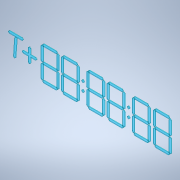
# Autodesk Inventor part: LED Clock Lights
Saved by Autodesk Inventor 2021 (Build 250183000, 183)
## iProperties
Created: 2020-06-27
Part Number: LED Clock Lights
Material: LED Bright
Document SubType Name: Modeling
Designer: dech3
Density: 1.188 g/cm^3
Appearance: Polycarbonate - Clear(2)
Author: dech3
Autodesk Inventor part; units mm, degrees
(part 1 of 2)
ref_plane "YZ Plane" through (0, 0, 0) normal (1, 0, 0) x (0, 1, 0)
ref_plane "XZ Plane" through (0, 0, 0) normal (0, 1, 0) x (-1, 0, 0)
ref_plane "XY Plane" through (0, 0, 0) normal (0, 0, 1) x (1, 0, 0)
sketch "Dot" plane through (0, 0, 0) normal (0, 0, 1) x (1, 0, 0)
  line L0 (-34.9663, 29.5091) -> (-32.9663, 29.5091)
  line L1 (-32.9663, 29.5091) -> (-29.7663, 26.3091)
  line L2 (-29.7663, 26.3091) -> (-29.7663, 24.3091)
  line L3 (-29.7663, 24.3091) -> (-32.9663, 21.1091)
  line L4 (-32.9663, 21.1091) -> (-34.9663, 21.1091)
  line L5 (-34.9663, 21.1091) -> (-38.1663, 24.3091)
  line L6 (-38.1663, 24.3091) -> (-38.1663, 26.3091)
  line L7 (-38.1663, 26.3091) -> (-34.9663, 29.5091)
  point P0 (-33.9663, 25.3091)
  dimension "d88" = 0
  dimension "d89" = 0
  dimension "d90" = 0
  dimension "d91" = 0
  dimension "d92" = 10
  dimension "d93" = 7.5
  dimension "d94" = 25
  dimension "d95" = 7.5
  dimension "d96" = 25
  dimension "d97" = 1.1
  dimension "d98" = 21
  dimension "d99" = 21
  dimension "d100" = 21
  dimension "d101" = 0
  dimension "d102" = 21
  dimension "d103" = 21
  dimension "d104" = 0
  dimension "d105" = 21
  dimension "d106" = 39
  dimension "d107" = 0
  dimension "d108" = 18
  dimension "d109" = 23
  dimension "d110" = 11.5
  dimension "d111" = 11.5
  dimension "d0" = 3.2
  dimension "d1" = 3.2
  dimension "d2" = 3.2
  dimension "d3" = 3.2
  dimension "d4" = 3.2
  dimension "d5" = 3.2
  dimension "d6" = 3.2
  dimension "d7" = 3.2
  dimension "d8" = 2
  dimension "d9" = 2
  dimension "d10" = 2
  dimension "d11" = 2
  measures "d0" horizontal distance of L1.end L0.end
  measures "d1" horizontal distance of L0.start L6.end
  measures "d2" horizontal distance of L0.start L6.end
  measures "d3" horizontal distance of L1.end L0.end
  measures "d4" horizontal distance of L4.end L5.end
  measures "d5" horizontal distance of L2.end L3.end
  measures "d6" horizontal distance of L2.end L3.end
  measures "d7" horizontal distance of L5.end L4.end
  measures "d8" distance of L1.end L2.end
  measures "d9" distance of L0.end L0.start
  measures "d10" distance of L3.end L4.end
  measures "d11" distance of L6.end L5.end
sketch "Slanted Segment Large" plane through (0, 0, 0) normal (0, 0, 1) x (1, 0, 0)
  line L0 (-252.8296, -124.6537) -> (-254.4296, -124.6537)
  line L1 (-254.4296, -124.6537) -> (-257.6296, -127.8537)
  line L2 (-257.6296, -127.8537) -> (-261.6917, -184.8537)
  line L3 (-253.6917, -184.8537) -> (-249.6296, -127.8537)
  line L4 (-249.6296, -127.8537) -> (-252.8296, -124.6537)
  line L5 (-261.6917, -184.8537) -> (-258.4917, -188.0537)
  line L6 (-258.4917, -188.0537) -> (-256.8917, -188.0537)
  line L7 (-256.8917, -188.0537) -> (-253.6917, -184.8537)
  point P0 (-253.3255, -154.094)
  point P1 (-253.6296, -124.6537)
  dimension "d88" = 0
  dimension "d89" = 0
  dimension "d90" = 0
  dimension "d91" = 0
  dimension "d92" = 10
  dimension "d93" = 7.5
  dimension "d94" = 25
  dimension "d95" = 7.5
  dimension "d96" = 25
  dimension "d97" = 1.1
  dimension "d98" = 21
  dimension "d99" = 21
  dimension "d100" = 21
  dimension "d101" = 0
  dimension "d102" = 21
  dimension "d103" = 21
  dimension "d104" = 0
  dimension "d105" = 21
  dimension "d106" = 39
  dimension "d107" = 0
  dimension "d108" = 18
  dimension "d109" = 23
  dimension "d110" = 11.5
  dimension "d111" = 11.5
  dimension "d12" = 3.2
  dimension "d13" = 3.2
  dimension "d14" = 8
  dimension "d15" = 3.2
  dimension "d16" = 3.2
  dimension "d17" = 57
  dimension "d18" = 3.2
  dimension "d19" = 3.2
  dimension "d20" = 3.2
  dimension "d21" = 3.2
  measures "d12" horizontal distance of L0.end L1.end
  measures "d13" horizontal distance of L3.end L0.start
  measures "d14" distance of L3.end L1.end
  measures "d15" horizontal distance of L3.end L0.start
  measures "d16" horizontal distance of L0.end L1.end
  measures "d17" vertical distance of L3.end L3.start
  measures "d18" horizontal distance of L5.end L2.end
  measures "d19" horizontal distance of L3.start L6.end
  measures "d20" horizontal distance of L2.end L5.end
  measures "d21" horizontal distance of L3.start L6.end
sketch "Single Segment" plane through (0, 0, 0) normal (0, 0, 1) x (1, 0, 0)
  arc A0 (130.9839, -3.9071) -> (131.691, -4.2) centre (131.691, -3.2) ccw
  arc A1 (131.691, 3.8) -> (130.9839, 3.5071) centre (131.691, 2.8) ccw
  line L0 (130.9839, -3.9071) -> (128.0768, -1)
  line L1 (128.0768, -0.2) -> (128.0768, 0.6)
  line L2 (128.0768, -0.2) -> (128.0768, -1)
  line L3 (130.9839, 3.5071) -> (128.0768, 0.6)
  line L4 (131.691, 3.8) -> (174.4626, 3.8)
  line L5 (174.4626, -4.2) -> (131.691, -4.2)
  arc A2 (175.1697, 3.5071) -> (174.4626, 3.8) centre (174.4626, 2.8) ccw
  arc A3 (174.4626, -4.2) -> (175.1697, -3.9071) centre (174.4626, -3.2) ccw
  line L6 (175.1697, -3.9071) -> (178.0768, -1)
  line L7 (178.0768, -0.2) -> (178.0768, -1)
  line L8 (178.0768, -0.2) -> (178.0768, 0.6)
  line L9 (175.1697, 3.5071) -> (178.0768, 0.6)
  point P0 (153.0768, 0)
  point P1 (131.2768, 3.8)
  point P2 (131.2768, -4.2)
  point P3 (174.8768, 3.8)
  point P4 (174.8768, -4.2)
  dimension "d88" = 0
  dimension "d89" = 0
  dimension "d90" = 0
  dimension "d91" = 0
  dimension "d92" = 10
  dimension "d93" = 7.5
  dimension "d94" = 25
  dimension "d95" = 7.5
  dimension "d96" = 25
  dimension "d97" = 1.1
  dimension "d98" = 21
  dimension "d99" = 21
  dimension "d100" = 21
  dimension "d101" = 0
  dimension "d102" = 21
  dimension "d103" = 21
  dimension "d104" = 0
  dimension "d105" = 21
  dimension "d106" = 39
  dimension "d107" = 0
  dimension "d108" = 18
  dimension "d109" = 23
  dimension "d110" = 11.5
  dimension "d111" = 11.5
  dimension "d22" = 3.2
  dimension "d23" = 3.2
  dimension "d24" = 3.2
  dimension "d25" = 3.2
  dimension "d26" = 3.2
  dimension "d27" = 3.2
  dimension "d28" = 3.2
  dimension "d29" = 1
  dimension "d30" = 8
  dimension "d31" = 8
  dimension "d32" = 3.2
  dimension "d33" = 3.2
  dimension "d34" = 50
  dimension "d35" = 135
  dimension "d36" = 50
  dimension "d37" = 135
  dimension "d38" = 4
  dimension "d39" = 4
  measures "d22" horizontal distance of point (131.277, -4.2) L0.end
  measures "d23" horizontal distance of L8.end point (174.877, 3.8)
  measures "d24" horizontal distance of point (131.277, 3.8) L1.end
  measures "d25" horizontal distance of L6.end point (174.877, -4.2)
  measures "d26" horizontal distance of L6.end point (174.877, -4.2)
  measures "d27" horizontal distance of point (131.277, 3.8) L1.end
  measures "d28" horizontal distance of point (131.277, -4.2) L0.end
  measures "d29" radius of A1
  measures "d30" distance of point (174.877, -4.2) point (174.877, 3.8)
  measures "d31" distance of point (131.277, -4.2) point (131.277, 3.8)
  measures "d32" horizontal distance of L8.end point (174.877, 3.8)
  measures "d33" horizontal distance of point (174.877, -4.2) L7.start
  measures "d34" distance of L7.start L1.start
  measures "d35" angle of L5 L6
  measures "d36" horizontal distance of L6.end L1.start
  measures "d37" angle of L4 L9
  measures "d38" vertical distance of L7.start point (174.877, -4.2)
  measures "d39" vertical distance of point (131.277, -4.2) L1.start
sketch "7 Segment Digit" plane through (0, 0, 0) normal (0, 0, 1) x (1, 0, 0)
  arc A0 (270.6071, -53.9929) -> (270.9, -53.2858) centre (269.9, -53.2858) ccw
  arc A1 (262.9, -53.2858) -> (263.1929, -53.9929) centre (263.9, -53.2858) ccw
  line L0 (270.6071, -53.9929) -> (267.7, -56.9)
  line L1 (266.9, -56.9) -> (266.1, -56.9)
  line L2 (266.9, -56.9) -> (267.7, -56.9)
  line L3 (263.1929, -53.9929) -> (266.1, -56.9)
  line L4 (262.9, -53.2858) -> (262.9, -10.5142)
  line L5 (270.9, -10.5142) -> (270.9, -53.2858)
  arc A2 (263.1929, -9.8071) -> (262.9, -10.5142) centre (263.9, -10.5142) ccw
  arc A3 (270.9, -10.5142) -> (270.6071, -9.8071) centre (269.9, -10.5142) ccw
  line L6 (270.6071, -9.8071) -> (267.7, -6.9)
  line L7 (266.9, -6.9) -> (267.7, -6.9)
  line L8 (266.9, -6.9) -> (266.1, -6.9)
  line L9 (263.1929, -9.8071) -> (266.1, -6.9)
  arc A4 (217.9071, -62.5071) -> (218.6142, -62.8) centre (218.6142, -61.8) ccw
  arc A5 (218.6142, -54.8) -> (217.9071, -55.0929) centre (218.6142, -55.8) ccw
  line L10 (217.9071, -62.5071) -> (215, -59.6)
  line L11 (215, -58.8) -> (215, -58)
  line L12 (215, -58.8) -> (215, -59.6)
  line L13 (217.9071, -55.0929) -> (215, -58)
  line L14 (218.6142, -54.8) -> (261.3858, -54.8)
  line L15 (261.3858, -62.8) -> (218.6142, -62.8)
  arc A6 (262.0929, -55.0929) -> (261.3858, -54.8) centre (261.3858, -55.8) ccw
  arc A7 (261.3858, -62.8) -> (262.0929, -62.5071) centre (261.3858, -61.8) ccw
  line L16 (262.0929, -62.5071) -> (265, -59.6)
  line L17 (265, -58.8) -> (265, -59.6)
  line L18 (265, -58.8) -> (265, -58)
  line L19 (262.0929, -55.0929) -> (265, -58)
  arc A8 (216.8071, -53.9929) -> (217.1, -53.2858) centre (216.1, -53.2858) ccw
  arc A9 (209.1, -53.2858) -> (209.3929, -53.9929) centre (210.1, -53.2858) ccw
  line L20 (216.8071, -53.9929) -> (213.9, -56.9)
  line L21 (213.1, -56.9) -> (212.3, -56.9)
  line L22 (213.1, -56.9) -> (213.9, -56.9)
  line L23 (209.3929, -53.9929) -> (212.3, -56.9)
  line L24 (209.1, -53.2858) -> (209.1, -10.5142)
  line L25 (217.1, -10.5142) -> (217.1, -53.2858)
  arc A10 (209.3929, -9.8071) -> (209.1, -10.5142) centre (210.1, -10.5142) ccw
  arc A11 (217.1, -10.5142) -> (216.8071, -9.8071) centre (216.1, -10.5142) ccw
  line L26 (216.8071, -9.8071) -> (213.9, -6.9)
  line L27 (213.1, -6.9) -> (213.9, -6.9)
  line L28 (213.1, -6.9) -> (212.3, -6.9)
  line L29 (209.3929, -9.8071) -> (212.3, -6.9)
  arc A12 (270.6071, -0.1929) -> (270.9, 0.5142) centre (269.9, 0.5142) ccw
  arc A13 (262.9, 0.5142) -> (263.1929, -0.1929) centre (263.9, 0.5142) ccw
  line L30 (270.6071, -0.1929) -> (267.7, -3.1)
  line L31 (266.9, -3.1) -> (266.1, -3.1)
  line L32 (266.9, -3.1) -> (267.7, -3.1)
  line L33 (263.1929, -0.1929) -> (266.1, -3.1)
  line L34 (262.9, 0.5142) -> (262.9, 43.2858)
  line L35 (270.9, 43.2858) -> (270.9, 0.5142)
  arc A14 (263.1929, 43.9929) -> (262.9, 43.2858) centre (263.9, 43.2858) ccw
  arc A15 (270.9, 43.2858) -> (270.6071, 43.9929) centre (269.9, 43.2858) ccw
  line L36 (270.6071, 43.9929) -> (267.7, 46.9)
  line L37 (266.9, 46.9) -> (267.7, 46.9)
  line L38 (266.9, 46.9) -> (266.1, 46.9)
  line L39 (263.1929, 43.9929) -> (266.1, 46.9)
  arc A16 (217.9071, -8.7071) -> (218.6142, -9) centre (218.6142, -8) ccw
  arc A17 (218.6142, -1) -> (217.9071, -1.2929) centre (218.6142, -2) ccw
  line L40 (217.9071, -8.7071) -> (215, -5.8)
  line L41 (215, -5) -> (215, -4.2)
  line L42 (215, -5) -> (215, -5.8)
  line L43 (217.9071, -1.2929) -> (215, -4.2)
  line L44 (218.6142, -1) -> (261.3858, -1)
  line L45 (261.3858, -9) -> (218.6142, -9)
  arc A18 (262.0929, -1.2929) -> (261.3858, -1) centre (261.3858, -2) ccw
  arc A19 (261.3858, -9) -> (262.0929, -8.7071) centre (261.3858, -8) ccw
  line L46 (262.0929, -8.7071) -> (265, -5.8)
  line L47 (265, -5) -> (265, -5.8)
  line L48 (265, -5) -> (265, -4.2)
  line L49 (262.0929, -1.2929) -> (265, -4.2)
  arc A20 (216.8071, -0.1929) -> (217.1, 0.5142) centre (216.1, 0.5142) ccw
  arc A21 (209.1, 0.5142) -> (209.3929, -0.1929) centre (210.1, 0.5142) ccw
  line L50 (216.8071, -0.1929) -> (213.9, -3.1)
  line L51 (213.1, -3.1) -> (212.3, -3.1)
  line L52 (213.1, -3.1) -> (213.9, -3.1)
  line L53 (209.3929, -0.1929) -> (212.3, -3.1)
  line L54 (209.1, 0.5142) -> (209.1, 43.2858)
  line L55 (217.1, 43.2858) -> (217.1, 0.5142)
  arc A22 (209.3929, 43.9929) -> (209.1, 43.2858) centre (210.1, 43.2858) ccw
  arc A23 (217.1, 43.2858) -> (216.8071, 43.9929) centre (216.1, 43.2858) ccw
  line L56 (216.8071, 43.9929) -> (213.9, 46.9)
  line L57 (213.1, 46.9) -> (213.9, 46.9)
  line L58 (213.1, 46.9) -> (212.3, 46.9)
  line L59 (209.3929, 43.9929) -> (212.3, 46.9)
  arc A24 (217.9071, 45.0929) -> (218.6142, 44.8) centre (218.6142, 45.8) ccw
  arc A25 (218.6142, 52.8) -> (217.9071, 52.5071) centre (218.6142, 51.8) ccw
  line L60 (217.9071, 45.0929) -> (215, 48)
  line L61 (215, 48.8) -> (215, 49.6)
  line L62 (215, 48.8) -> (215, 48)
  line L63 (217.9071, 52.5071) -> (215, 49.6)
  line L64 (218.6142, 52.8) -> (261.3858, 52.8)
  line L65 (261.3858, 44.8) -> (218.6142, 44.8)
  arc A26 (262.0929, 52.5071) -> (261.3858, 52.8) centre (261.3858, 51.8) ccw
  arc A27 (261.3858, 44.8) -> (262.0929, 45.0929) centre (261.3858, 45.8) ccw
  line L66 (262.0929, 45.0929) -> (265, 48)
  line L67 (265, 48.8) -> (265, 48)
  line L68 (265, 48.8) -> (265, 49.6)
  line L69 (262.0929, 52.5071) -> (265, 49.6)
  point P0 (239.8857, -4.9143)
  dimension "d40" = 1.1
  dimension "d41" = 1.1
  dimension "d42" = 1.1
  dimension "d43" = 1.1
  dimension "d44" = 1.1
  dimension "d45" = 1.1
  dimension "d46" = 1.1
  dimension "d47" = 1.1
  dimension "d48" = 1.1
  dimension "d49" = 1.1
  dimension "d50" = 1.1
  dimension "d51" = 1.1
  dimension "d52" = 1.1
  dimension "d53" = 1.1
  dimension "d54" = 1.1
  dimension "d55" = 1.1
  dimension "d88" = 0
  dimension "d89" = 0
  dimension "d90" = 0
  dimension "d91" = 0
  dimension "d92" = 10
  dimension "d93" = 7.5
  dimension "d94" = 25
  dimension "d95" = 7.5
sketch "+ sign" plane through (0, 0, 0) normal (0, 0, 1) x (1, 0, 0)
  arc A0 (-229.4607, -27.8865) -> (-229.1679, -28.5937) centre (-228.4607, -27.8865) ccw
  arc A1 (-221.7536, -28.5937) -> (-221.4607, -27.8865) centre (-222.4607, -27.8865) ccw
  arc A2 (-247.3536, -10.4079) -> (-246.6465, -10.7008) centre (-246.6465, -9.7008) ccw
  arc A3 (-229.1679, 15.1921) -> (-229.4607, 14.485) centre (-228.4607, 14.485) ccw
  arc A4 (-221.4607, 14.485) -> (-221.7536, 15.1921) centre (-222.4607, 14.485) ccw
  arc A5 (-203.5679, -2.9937) -> (-204.275, -2.7008) centre (-204.275, -3.7008) ccw
  arc A6 (-204.275, -10.7008) -> (-203.5679, -10.4079) centre (-204.275, -9.7008) ccw
  line L0 (-247.3536, -10.4079) -> (-250.2607, -7.5008)
  line L1 (-229.1679, -28.5937) -> (-226.2607, -31.5008)
  line L2 (-203.5679, -10.4079) -> (-200.6607, -7.5008)
  line L3 (-221.4607, -2.7008) -> (-221.4607, 14.485)
  line L4 (-221.7536, 15.1921) -> (-224.6607, 18.0992)
  line L5 (-224.6607, 18.0992) -> (-226.2607, 18.0992)
  line L6 (-204.275, -2.7008) -> (-221.4607, -2.7008)
  line L7 (-203.5679, -2.9937) -> (-200.6607, -5.9008)
  line L8 (-200.6607, -5.9008) -> (-200.6607, -7.5008)
  line L9 (-204.275, -10.7008) -> (-221.4607, -10.7008)
  line L10 (-221.4607, -27.8865) -> (-221.4607, -10.7008)
  line L11 (-226.2607, 18.0992) -> (-229.1679, 15.1921)
  arc A7 (-246.6465, -2.7008) -> (-247.3536, -2.9937) centre (-246.6465, -3.7008) ccw
  line L12 (-229.4607, 14.485) -> (-229.4607, -2.7008)
  line L13 (-246.6465, -2.7008) -> (-229.4607, -2.7008)
  line L14 (-247.3536, -2.9937) -> (-250.2607, -5.9008)
  line L15 (-250.2607, -5.9008) -> (-250.2607, -7.5008)
  line L16 (-246.6465, -10.7008) -> (-229.4607, -10.7008)
  line L17 (-229.4607, -10.7008) -> (-229.4607, -27.8865)
  line L18 (-226.2607, -31.5008) -> (-224.6607, -31.5008)
  line L19 (-224.6607, -31.5008) -> (-221.7536, -28.5937)
  point P0 (-225.4266, -6.7349)
  point P1 (-221.4607, 14.8992)
  point P2 (-203.8607, -2.7008)
  point P3 (-203.8607, -10.7008)
  point P4 (-229.4607, 14.8992)
  point P5 (-247.0607, -2.7008)
  point P6 (-247.0607, -10.7008)
  point P7 (-229.4607, -28.3008)
  point P8 (-221.4607, -28.3008)
  dimension "d88" = 0
  dimension "d89" = 0
  dimension "d90" = 0
  dimension "d91" = 0
  dimension "d92" = 10
  dimension "d93" = 7.5
  dimension "d94" = 25
  dimension "d95" = 7.5
  dimension "d96" = 25
  dimension "d97" = 1.1
  dimension "d98" = 21
  dimension "d99" = 21
  dimension "d100" = 21
  dimension "d101" = 0
  dimension "d102" = 21
  dimension "d103" = 21
  dimension "d104" = 0
  dimension "d105" = 21
  dimension "d106" = 39
  dimension "d107" = 0
  dimension "d108" = 18
  dimension "d109" = 23
  dimension "d110" = 11.5
  dimension "d111" = 11.5
  dimension "d56" = 3.2
  dimension "d57" = 3.2
  dimension "d58" = 3.2
  dimension "d59" = 3.2
  dimension "d60" = 3.2
  dimension "d61" = 3.2
  dimension "d62" = 3.2
  dimension "d63" = 3.2
  dimension "d64" = 3.2
  dimension "d65" = 3.2
  dimension "d66" = 3.2
  dimension "d67" = 3.2
  dimension "d68" = 3.2
  dimension "d69" = 0
  dimension "d70" = 0
  dimension "d71" = 8
  dimension "d72" = 8
  dimension "d73" = 0
  dimension "d74" = 0
  dimension "d75" = 3.2
  dimension "d76" = 3.2
  dimension "d77" = 3.2
  dimension "d78" = 90
  dimension "d79" = 17.6
  dimension "d80" = 17.6
  dimension "d81" = 17.6
  dimension "d82" = 17.6
  dimension "d83" = 17.6
  dimension "d84" = 0
  dimension "d85" = 17.6
  dimension "d86" = 1
  dimension "d87" = 1
  measures "d56" distance from line of point (-247.061, -2.701) L15
  measures "d57" horizontal distance of point (-247.061, -2.701) L14.end
  measures "d58" horizontal distance of point (-247.061, -10.701) L0.end
  measures "d59" horizontal distance of point (-247.061, -10.701) L0.end
  measures "d60" horizontal distance of L1.end point (-229.461, -28.301)
  measures "d61" horizontal distance of point (-229.461, -28.301) L1.end
  measures "d62" horizontal distance of point (-221.461, -28.301) L18.end
  measures "d63" horizontal distance of L18.end point (-221.461, -28.301)
  measures "d64" horizontal distance of L2.end point (-203.861, -10.701)
  measures "d65" horizontal distance of point (-203.861, -10.701) L2.end
  measures "d66" horizontal distance of point (-203.861, -2.701) L7.end
  measures "d67" horizontal distance of point (-203.861, -2.701) L7.end
  measures "d68" horizontal distance of L4.end point (-221.461, 14.899)
  measures "d69" distance between parallel lines of L3 L10
  measures "d70" distance between parallel lines of L12 L17
  measures "d71" distance between parallel lines of L3 L12
  measures "d72" distance between parallel lines of L16 L13
  measures "d73" distance between parallel lines of L13 L6
  measures "d74" distance between parallel lines of L16 L9
  measures "d75" horizontal distance of L5.end point (-229.461, 14.899)
  measures "d76" horizontal distance of L5.end point (-229.461, 14.899)
  measures "d77" horizontal distance of L4.end point (-221.461, 14.899)
  measures "d78" angle of L6 L3
  measures "d79" distance of L12.end point (-247.061, -2.701)
  measures "d80" distance of point (-203.861, -2.701) L3.start
  measures "d81" distance of point (-221.461, 14.899) L3.start
  measures "d82" distance of point (-221.461, -28.301) L10.end
  measures "d83" distance of point (-229.461, -28.301) L16.end
  measures "d84" distance of L10.end L9.end
  measures "d85" distance of L10.end point (-203.861, -10.701)
  measures "d86" radius of A3
  measures "d87" radius of A0
sketch "Clock Face with T +-" plane through (0, 0, 0) normal (0, 0, 1) x (1, 0, 0)
  line L0 (121.9, 15) -> (123.9, 15)
  line L1 (123.9, 15) -> (127.1, 11.8)
  line L2 (127.1, 11.8) -> (127.1, 9.8)
  line L3 (127.1, 9.8) -> (123.9, 6.6)
  line L4 (123.9, 6.6) -> (121.9, 6.6)
  line L5 (121.9, 6.6) -> (118.7, 9.8)
  line L6 (118.7, 9.8) -> (118.7, 11.8)
  line L7 (118.7, 11.8) -> (121.9, 15)
  line L8 (121.9, -14.4) -> (123.9, -14.4)
  line L9 (123.9, -14.4) -> (127.1, -17.6)
  line L10 (127.1, -17.6) -> (127.1, -19.6)
  line L11 (127.1, -19.6) -> (123.9, -22.8)
  line L12 (123.9, -22.8) -> (121.9, -22.8)
  line L13 (121.9, -22.8) -> (118.7, -19.6)
  line L14 (118.7, -19.6) -> (118.7, -17.6)
  line L15 (118.7, -17.6) -> (121.9, -14.4)
  line L16 (-34.2, 15) -> (-32.2, 15)
  line L17 (-32.2, 15) -> (-29, 11.8)
  line L18 (-29, 11.8) -> (-29, 9.8)
  line L19 (-29, 9.8) -> (-32.2, 6.6)
  line L20 (-32.2, 6.6) -> (-34.2, 6.6)
  line L21 (-34.2, 6.6) -> (-37.4, 9.8)
  line L22 (-37.4, 9.8) -> (-37.4, 11.8)
  line L23 (-37.4, 11.8) -> (-34.2, 15)
  line L24 (-34.2, -14.4) -> (-32.2, -14.4)
  line L25 (-32.2, -14.4) -> (-29, -17.6)
  line L26 (-29, -17.6) -> (-29, -19.6)
  line L27 (-29, -19.6) -> (-32.2, -22.8)
  line L28 (-32.2, -22.8) -> (-34.2, -22.8)
  line L29 (-34.2, -22.8) -> (-37.4, -19.6)
  line L30 (-37.4, -19.6) -> (-37.4, -17.6)
  line L31 (-37.4, -17.6) -> (-34.2, -14.4)
  line L32 (-262.2, 25.9) -> (-263.8, 25.9)
  line L33 (-263.8, 25.9) -> (-267, 22.7)
  line L34 (-267, 22.7) -> (-271.0621, -34.3)
  line L35 (-263.0621, -34.3) -> (-259, 22.7)
  line L36 (-259, 22.7) -> (-262.2, 25.9)
  line L37 (-271.0621, -34.3) -> (-267.8621, -37.5)
  line L38 (-267.8621, -37.5) -> (-266.2621, -37.5)
  line L39 (-266.2621, -37.5) -> (-263.0621, -34.3)
  arc A0 (268.7071, -52.7929) -> (269, -52.0858) centre (268, -52.0858) ccw
  arc A1 (261, -52.0858) -> (261.2929, -52.7929) centre (262, -52.0858) ccw
  line L40 (268.7071, -52.7929) -> (265.8, -55.7)
  line L41 (265, -55.7) -> (264.2, -55.7)
  line L42 (265, -55.7) -> (265.8, -55.7)
  line L43 (261.2929, -52.7929) -> (264.2, -55.7)
  line L44 (261, -52.0858) -> (261, -9.3142)
  line L45 (269, -9.3142) -> (269, -52.0858)
  arc A2 (261.2929, -8.6071) -> (261, -9.3142) centre (262, -9.3142) ccw
  arc A3 (269, -9.3142) -> (268.7071, -8.6071) centre (268, -9.3142) ccw
  line L46 (268.7071, -8.6071) -> (265.8, -5.7)
  line L47 (265, -5.7) -> (265.8, -5.7)
  line L48 (265, -5.7) -> (264.2, -5.7)
  line L49 (261.2929, -8.6071) -> (264.2, -5.7)
  arc A4 (216.0071, -61.3071) -> (216.7142, -61.6) centre (216.7142, -60.6) ccw
  arc A5 (216.7142, -53.6) -> (216.0071, -53.8929) centre (216.7142, -54.6) ccw
  line L50 (216.0071, -61.3071) -> (213.1, -58.4)
  line L51 (213.1, -57.6) -> (213.1, -56.8)
  line L52 (213.1, -57.6) -> (213.1, -58.4)
  line L53 (216.0071, -53.8929) -> (213.1, -56.8)
  line L54 (216.7142, -53.6) -> (259.4858, -53.6)
  line L55 (259.4858, -61.6) -> (216.7142, -61.6)
  arc A6 (260.1929, -53.8929) -> (259.4858, -53.6) centre (259.4858, -54.6) ccw
  arc A7 (259.4858, -61.6) -> (260.1929, -61.3071) centre (259.4858, -60.6) ccw
  line L56 (260.1929, -61.3071) -> (263.1, -58.4)
  line L57 (263.1, -57.6) -> (263.1, -58.4)
  line L58 (263.1, -57.6) -> (263.1, -56.8)
  line L59 (260.1929, -53.8929) -> (263.1, -56.8)
  arc A8 (214.9071, -52.7929) -> (215.2, -52.0858) centre (214.2, -52.0858) ccw
  arc A9 (207.2, -52.0858) -> (207.4929, -52.7929) centre (208.2, -52.0858) ccw
  line L60 (214.9071, -52.7929) -> (212, -55.7)
  line L61 (211.2, -55.7) -> (210.4, -55.7)
  line L62 (211.2, -55.7) -> (212, -55.7)
  line L63 (207.4929, -52.7929) -> (210.4, -55.7)
  line L64 (207.2, -52.0858) -> (207.2, -9.3142)
  line L65 (215.2, -9.3142) -> (215.2, -52.0858)
  arc A10 (207.4929, -8.6071) -> (207.2, -9.3142) centre (208.2, -9.3142) ccw
  arc A11 (215.2, -9.3142) -> (214.9071, -8.6071) centre (214.2, -9.3142) ccw
  line L66 (214.9071, -8.6071) -> (212, -5.7)
  line L67 (211.2, -5.7) -> (212, -5.7)
  line L68 (211.2, -5.7) -> (210.4, -5.7)
  line L69 (207.4929, -8.6071) -> (210.4, -5.7)
  arc A12 (268.7071, 1.0071) -> (269, 1.7142) centre (268, 1.7142) ccw
  arc A13 (261, 1.7142) -> (261.2929, 1.0071) centre (262, 1.7142) ccw
  line L70 (268.7071, 1.0071) -> (265.8, -1.9)
  line L71 (265, -1.9) -> (264.2, -1.9)
  line L72 (265, -1.9) -> (265.8, -1.9)
  line L73 (261.2929, 1.0071) -> (264.2, -1.9)
  line L74 (261, 1.7142) -> (261, 44.4858)
  line L75 (269, 44.4858) -> (269, 1.7142)
  arc A14 (261.2929, 45.1929) -> (261, 44.4858) centre (262, 44.4858) ccw
  arc A15 (269, 44.4858) -> (268.7071, 45.1929) centre (268, 44.4858) ccw
  line L76 (268.7071, 45.1929) -> (265.8, 48.1)
  line L77 (265, 48.1) -> (265.8, 48.1)
  line L78 (265, 48.1) -> (264.2, 48.1)
  line L79 (261.2929, 45.1929) -> (264.2, 48.1)
  arc A16 (216.0071, -7.5071) -> (216.7142, -7.8) centre (216.7142, -6.8) ccw
  arc A17 (216.7142, 0.2) -> (216.0071, -0.0929) centre (216.7142, -0.8) ccw
  line L80 (216.0071, -7.5071) -> (213.1, -4.6)
  line L81 (213.1, -3.8) -> (213.1, -3)
  line L82 (213.1, -3.8) -> (213.1, -4.6)
  line L83 (216.0071, -0.0929) -> (213.1, -3)
  line L84 (216.7142, 0.2) -> (259.4858, 0.2)
  line L85 (259.4858, -7.8) -> (216.7142, -7.8)
  arc A18 (260.1929, -0.0929) -> (259.4858, 0.2) centre (259.4858, -0.8) ccw
  arc A19 (259.4858, -7.8) -> (260.1929, -7.5071) centre (259.4858, -6.8) ccw
  line L86 (260.1929, -7.5071) -> (263.1, -4.6)
  line L87 (263.1, -3.8) -> (263.1, -4.6)
  line L88 (263.1, -3.8) -> (263.1, -3)
  line L89 (260.1929, -0.0929) -> (263.1, -3)
  arc A20 (214.9071, 1.0071) -> (215.2, 1.7142) centre (214.2, 1.7142) ccw
  arc A21 (207.2, 1.7142) -> (207.4929, 1.0071) centre (208.2, 1.7142) ccw
  line L90 (214.9071, 1.0071) -> (212, -1.9)
  line L91 (211.2, -1.9) -> (210.4, -1.9)
  line L92 (211.2, -1.9) -> (212, -1.9)
  line L93 (207.4929, 1.0071) -> (210.4, -1.9)
  line L94 (207.2, 1.7142) -> (207.2, 44.4858)
  line L95 (215.2, 44.4858) -> (215.2, 1.7142)
  arc A22 (207.4929, 45.1929) -> (207.2, 44.4858) centre (208.2, 44.4858) ccw
  arc A23 (215.2, 44.4858) -> (214.9071, 45.1929) centre (214.2, 44.4858) ccw
  line L96 (214.9071, 45.1929) -> (212, 48.1)
  line L97 (211.2, 48.1) -> (212, 48.1)
  line L98 (211.2, 48.1) -> (210.4, 48.1)
  line L99 (207.4929, 45.1929) -> (210.4, 48.1)
  arc A24 (216.0071, 46.2929) -> (216.7142, 46) centre (216.7142, 47) ccw
  arc A25 (216.7142, 54) -> (216.0071, 53.7071) centre (216.7142, 53) ccw
  line L100 (216.0071, 46.2929) -> (213.1, 49.2)
  line L101 (213.1, 50) -> (213.1, 50.8)
  line L102 (213.1, 50) -> (213.1, 49.2)
  line L103 (216.0071, 53.7071) -> (213.1, 50.8)
  line L104 (216.7142, 54) -> (259.4858, 54)
  line L105 (259.4858, 46) -> (216.7142, 46)
  arc A26 (260.1929, 53.7071) -> (259.4858, 54) centre (259.4858, 53) ccw
  arc A27 (259.4858, 46) -> (260.1929, 46.2929) centre (259.4858, 47) ccw
  line L106 (260.1929, 46.2929) -> (263.1, 49.2)
  line L107 (263.1, 50) -> (263.1, 49.2)
  line L108 (263.1, 50) -> (263.1, 50.8)
  line L109 (260.1929, 53.7071) -> (263.1, 50.8)
  arc A28 (-285.0929, 27.2929) -> (-284.3858, 27) centre (-284.3858, 28) ccw
  arc A29 (-284.3858, 35) -> (-285.0929, 34.7071) centre (-284.3858, 34) ccw
  line L110 (-285.0929, 27.2929) -> (-288, 30.2)
  line L111 (-288, 31) -> (-288, 31.8)
  line L112 (-288, 31) -> (-288, 30.2)
  line L113 (-285.0929, 34.7071) -> (-288, 31.8)
  line L114 (-284.3858, 35) -> (-241.6142, 35)
  line L115 (-241.6142, 27) -> (-284.3858, 27)
  arc A30 (-240.9071, 34.7071) -> (-241.6142, 35) centre (-241.6142, 34) ccw
  arc A31 (-241.6142, 27) -> (-240.9071, 27.2929) centre (-241.6142, 28) ccw
  line L116 (-240.9071, 27.2929) -> (-238, 30.2)
  line L117 (-238, 31) -> (-238, 30.2)
  line L118 (-238, 31) -> (-238, 31.8)
  line L119 (-240.9071, 34.7071) -> (-238, 31.8)
  arc A32 (196.9071, -52.7929) -> (197.2, -52.0858) centre (196.2, -52.0858) ccw
  arc A33 (189.2, -52.0858) -> (189.4929, -52.7929) centre (190.2, -52.0858) ccw
  line L120 (196.9071, -52.7929) -> (194, -55.7)
  line L121 (193.2, -55.7) -> (192.4, -55.7)
  line L122 (193.2, -55.7) -> (194, -55.7)
  line L123 (189.4929, -52.7929) -> (192.4, -55.7)
  line L124 (189.2, -52.0858) -> (189.2, -9.3142)
  line L125 (197.2, -9.3142) -> (197.2, -52.0858)
  arc A34 (189.4929, -8.6071) -> (189.2, -9.3142) centre (190.2, -9.3142) ccw
  arc A35 (197.2, -9.3142) -> (196.9071, -8.6071) centre (196.2, -9.3142) ccw
  line L126 (196.9071, -8.6071) -> (194, -5.7)
  line L127 (193.2, -5.7) -> (194, -5.7)
  line L128 (193.2, -5.7) -> (192.4, -5.7)
  line L129 (189.4929, -8.6071) -> (192.4, -5.7)
  arc A36 (144.2071, -61.3071) -> (144.9142, -61.6) centre (144.9142, -60.6) ccw
  arc A37 (144.9142, -53.6) -> (144.2071, -53.8929) centre (144.9142, -54.6) ccw
  line L130 (144.2071, -61.3071) -> (141.3, -58.4)
  line L131 (141.3, -57.6) -> (141.3, -56.8)
  line L132 (141.3, -57.6) -> (141.3, -58.4)
  line L133 (144.2071, -53.8929) -> (141.3, -56.8)
  line L134 (144.9142, -53.6) -> (187.6858, -53.6)
  line L135 (187.6858, -61.6) -> (144.9142, -61.6)
  arc A38 (188.3929, -53.8929) -> (187.6858, -53.6) centre (187.6858, -54.6) ccw
  arc A39 (187.6858, -61.6) -> (188.3929, -61.3071) centre (187.6858, -60.6) ccw
  line L136 (188.3929, -61.3071) -> (191.3, -58.4)
  line L137 (191.3, -57.6) -> (191.3, -58.4)
  line L138 (191.3, -57.6) -> (191.3, -56.8)
  line L139 (188.3929, -53.8929) -> (191.3, -56.8)
  arc A40 (143.1071, -52.7929) -> (143.4, -52.0858) centre (142.4, -52.0858) ccw
  arc A41 (135.4, -52.0858) -> (135.6929, -52.7929) centre (136.4, -52.0858) ccw
  line L140 (143.1071, -52.7929) -> (140.2, -55.7)
  line L141 (139.4, -55.7) -> (138.6, -55.7)
  line L142 (139.4, -55.7) -> (140.2, -55.7)
  line L143 (135.6929, -52.7929) -> (138.6, -55.7)
  line L144 (135.4, -52.0858) -> (135.4, -9.3142)
  line L145 (143.4, -9.3142) -> (143.4, -52.0858)
  arc A42 (135.6929, -8.6071) -> (135.4, -9.3142) centre (136.4, -9.3142) ccw
  arc A43 (143.4, -9.3142) -> (143.1071, -8.6071) centre (142.4, -9.3142) ccw
  line L146 (143.1071, -8.6071) -> (140.2, -5.7)
  line L147 (139.4, -5.7) -> (140.2, -5.7)
  line L148 (139.4, -5.7) -> (138.6, -5.7)
  line L149 (135.6929, -8.6071) -> (138.6, -5.7)
  arc A44 (196.9071, 1.0071) -> (197.2, 1.7142) centre (196.2, 1.7142) ccw
  arc A45 (189.2, 1.7142) -> (189.4929, 1.0071) centre (190.2, 1.7142) ccw
  line L150 (196.9071, 1.0071) -> (194, -1.9)
  line L151 (193.2, -1.9) -> (192.4, -1.9)
  line L152 (193.2, -1.9) -> (194, -1.9)
  line L153 (189.4929, 1.0071) -> (192.4, -1.9)
  line L154 (189.2, 1.7142) -> (189.2, 44.4858)
  line L155 (197.2, 44.4858) -> (197.2, 1.7142)
  arc A46 (189.4929, 45.1929) -> (189.2, 44.4858) centre (190.2, 44.4858) ccw
  arc A47 (197.2, 44.4858) -> (196.9071, 45.1929) centre (196.2, 44.4858) ccw
  line L156 (196.9071, 45.1929) -> (194, 48.1)
  line L157 (193.2, 48.1) -> (194, 48.1)
  line L158 (193.2, 48.1) -> (192.4, 48.1)
  line L159 (189.4929, 45.1929) -> (192.4, 48.1)
  arc A48 (144.2071, -7.5071) -> (144.9142, -7.8) centre (144.9142, -6.8) ccw
  arc A49 (144.9142, 0.2) -> (144.2071, -0.0929) centre (144.9142, -0.8) ccw
  line L160 (144.2071, -7.5071) -> (141.3, -4.6)
  line L161 (141.3, -3.8) -> (141.3, -3)
  line L162 (141.3, -3.8) -> (141.3, -4.6)
  line L163 (144.2071, -0.0929) -> (141.3, -3)
  line L164 (144.9142, 0.2) -> (187.6858, 0.2)
  line L165 (187.6858, -7.8) -> (144.9142, -7.8)
  arc A50 (188.3929, -0.0929) -> (187.6858, 0.2) centre (187.6858, -0.8) ccw
  arc A51 (187.6858, -7.8) -> (188.3929, -7.5071) centre (187.6858, -6.8) ccw
  line L166 (188.3929, -7.5071) -> (191.3, -4.6)
  line L167 (191.3, -3.8) -> (191.3, -4.6)
  line L168 (191.3, -3.8) -> (191.3, -3)
  line L169 (188.3929, -0.0929) -> (191.3, -3)
  arc A52 (143.1071, 1.0071) -> (143.4, 1.7142) centre (142.4, 1.7142) ccw
  arc A53 (135.4, 1.7142) -> (135.6929, 1.0071) centre (136.4, 1.7142) ccw
  line L170 (143.1071, 1.0071) -> (140.2, -1.9)
  line L171 (139.4, -1.9) -> (138.6, -1.9)
  line L172 (139.4, -1.9) -> (140.2, -1.9)
  line L173 (135.6929, 1.0071) -> (138.6, -1.9)
  line L174 (135.4, 1.7142) -> (135.4, 44.4858)
  line L175 (143.4, 44.4858) -> (143.4, 1.7142)
  arc A54 (135.6929, 45.1929) -> (135.4, 44.4858) centre (136.4, 44.4858) ccw
  arc A55 (143.4, 44.4858) -> (143.1071, 45.1929) centre (142.4, 44.4858) ccw
  line L176 (143.1071, 45.1929) -> (140.2, 48.1)
  line L177 (139.4, 48.1) -> (140.2, 48.1)
  line L178 (139.4, 48.1) -> (138.6, 48.1)
  line L179 (135.6929, 45.1929) -> (138.6, 48.1)
  arc A56 (144.2071, 46.2929) -> (144.9142, 46) centre (144.9142, 47) ccw
  arc A57 (144.9142, 54) -> (144.2071, 53.7071) centre (144.9142, 53) ccw
  line L180 (144.2071, 46.2929) -> (141.3, 49.2)
  line L181 (141.3, 50) -> (141.3, 50.8)
  line L182 (141.3, 50) -> (141.3, 49.2)
  line L183 (144.2071, 53.7071) -> (141.3, 50.8)
  line L184 (144.9142, 54) -> (187.6858, 54)
  line L185 (187.6858, 46) -> (144.9142, 46)
  arc A58 (188.3929, 53.7071) -> (187.6858, 54) centre (187.6858, 53) ccw
  arc A59 (187.6858, 46) -> (188.3929, 46.2929) centre (187.6858, 47) ccw
  line L186 (188.3929, 46.2929) -> (191.3, 49.2)
  line L187 (191.3, 50) -> (191.3, 49.2)
  line L188 (191.3, 50) -> (191.3, 50.8)
  line L189 (188.3929, 53.7071) -> (191.3, 50.8)
  arc A60 (110.1071, -52.7929) -> (110.4, -52.0858) centre (109.4, -52.0858) ccw
  arc A61 (102.4, -52.0858) -> (102.6929, -52.7929) centre (103.4, -52.0858) ccw
  line L190 (110.1071, -52.7929) -> (107.2, -55.7)
  line L191 (106.4, -55.7) -> (105.6, -55.7)
  line L192 (106.4, -55.7) -> (107.2, -55.7)
  line L193 (102.6929, -52.7929) -> (105.6, -55.7)
  line L194 (102.4, -52.0858) -> (102.4, -9.3142)
  line L195 (110.4, -9.3142) -> (110.4, -52.0858)
  arc A62 (102.6929, -8.6071) -> (102.4, -9.3142) centre (103.4, -9.3142) ccw
  arc A63 (110.4, -9.3142) -> (110.1071, -8.6071) centre (109.4, -9.3142) ccw
  line L196 (110.1071, -8.6071) -> (107.2, -5.7)
  line L197 (106.4, -5.7) -> (107.2, -5.7)
  line L198 (106.4, -5.7) -> (105.6, -5.7)
  line L199 (102.6929, -8.6071) -> (105.6, -5.7)
  arc A64 (57.4071, -61.3071) -> (58.1142, -61.6) centre (58.1142, -60.6) ccw
  arc A65 (58.1142, -53.6) -> (57.4071, -53.8929) centre (58.1142, -54.6) ccw
  line L200 (57.4071, -61.3071) -> (54.5, -58.4)
  line L201 (54.5, -57.6) -> (54.5, -56.8)
  line L202 (54.5, -57.6) -> (54.5, -58.4)
  line L203 (57.4071, -53.8929) -> (54.5, -56.8)
  line L204 (58.1142, -53.6) -> (100.8858, -53.6)
  line L205 (100.8858, -61.6) -> (58.1142, -61.6)
  arc A66 (101.5929, -53.8929) -> (100.8858, -53.6) centre (100.8858, -54.6) ccw
  arc A67 (100.8858, -61.6) -> (101.5929, -61.3071) centre (100.8858, -60.6) ccw
  line L206 (101.5929, -61.3071) -> (104.5, -58.4)
  line L207 (104.5, -57.6) -> (104.5, -58.4)
  line L208 (104.5, -57.6) -> (104.5, -56.8)
  line L209 (101.5929, -53.8929) -> (104.5, -56.8)
  arc A68 (56.3071, -52.7929) -> (56.6, -52.0858) centre (55.6, -52.0858) ccw
  arc A69 (48.6, -52.0858) -> (48.8929, -52.7929) centre (49.6, -52.0858) ccw
  line L210 (56.3071, -52.7929) -> (53.4, -55.7)
  line L211 (52.6, -55.7) -> (51.8, -55.7)
  line L212 (52.6, -55.7) -> (53.4, -55.7)
  line L213 (48.8929, -52.7929) -> (51.8, -55.7)
  line L214 (48.6, -52.0858) -> (48.6, -9.3142)
  line L215 (56.6, -9.3142) -> (56.6, -52.0858)
  arc A70 (48.8929, -8.6071) -> (48.6, -9.3142) centre (49.6, -9.3142) ccw
  arc A71 (56.6, -9.3142) -> (56.3071, -8.6071) centre (55.6, -9.3142) ccw
  line L216 (56.3071, -8.6071) -> (53.4, -5.7)
  line L217 (52.6, -5.7) -> (53.4, -5.7)
  line L218 (52.6, -5.7) -> (51.8, -5.7)
  line L219 (48.8929, -8.6071) -> (51.8, -5.7)
  arc A72 (110.1071, 1.0071) -> (110.4, 1.7142) centre (109.4, 1.7142) ccw
  arc A73 (102.4, 1.7142) -> (102.6929, 1.0071) centre (103.4, 1.7142) ccw
  line L220 (110.1071, 1.0071) -> (107.2, -1.9)
  line L221 (106.4, -1.9) -> (105.6, -1.9)
  line L222 (106.4, -1.9) -> (107.2, -1.9)
  line L223 (102.6929, 1.0071) -> (105.6, -1.9)
  line L224 (102.4, 1.7142) -> (102.4, 44.4858)
  line L225 (110.4, 44.4858) -> (110.4, 1.7142)
  arc A74 (102.6929, 45.1929) -> (102.4, 44.4858) centre (103.4, 44.4858) ccw
  arc A75 (110.4, 44.4858) -> (110.1071, 45.1929) centre (109.4, 44.4858) ccw
  line L226 (110.1071, 45.1929) -> (107.2, 48.1)
  line L227 (106.4, 48.1) -> (107.2, 48.1)
  line L228 (106.4, 48.1) -> (105.6, 48.1)
  line L229 (102.6929, 45.1929) -> (105.6, 48.1)
  arc A76 (57.4071, -7.5071) -> (58.1142, -7.8) centre (58.1142, -6.8) ccw
  arc A77 (58.1142, 0.2) -> (57.4071, -0.0929) centre (58.1142, -0.8) ccw
  line L230 (57.4071, -7.5071) -> (54.5, -4.6)
  line L231 (54.5, -3.8) -> (54.5, -3)
  line L232 (54.5, -3.8) -> (54.5, -4.6)
  line L233 (57.4071, -0.0929) -> (54.5, -3)
  line L234 (58.1142, 0.2) -> (100.8858, 0.2)
  line L235 (100.8858, -7.8) -> (58.1142, -7.8)
  arc A78 (101.5929, -0.0929) -> (100.8858, 0.2) centre (100.8858, -0.8) ccw
  arc A79 (100.8858, -7.8) -> (101.5929, -7.5071) centre (100.8858, -6.8) ccw
  line L236 (101.5929, -7.5071) -> (104.5, -4.6)
  line L237 (104.5, -3.8) -> (104.5, -4.6)
  line L238 (104.5, -3.8) -> (104.5, -3)
  line L239 (101.5929, -0.0929) -> (104.5, -3)
  arc A80 (56.3071, 1.0071) -> (56.6, 1.7142) centre (55.6, 1.7142) ccw
  arc A81 (48.6, 1.7142) -> (48.8929, 1.0071) centre (49.6, 1.7142) ccw
  line L240 (56.3071, 1.0071) -> (53.4, -1.9)
  line L241 (52.6, -1.9) -> (51.8, -1.9)
  line L242 (52.6, -1.9) -> (53.4, -1.9)
  line L243 (48.8929, 1.0071) -> (51.8, -1.9)
  line L244 (48.6, 1.7142) -> (48.6, 44.4858)
  line L245 (56.6, 44.4858) -> (56.6, 1.7142)
  arc A82 (48.8929, 45.1929) -> (48.6, 44.4858) centre (49.6, 44.4858) ccw
  arc A83 (56.6, 44.4858) -> (56.3071, 45.1929) centre (55.6, 44.4858) ccw
  line L246 (56.3071, 45.1929) -> (53.4, 48.1)
  line L247 (52.6, 48.1) -> (53.4, 48.1)
  line L248 (52.6, 48.1) -> (51.8, 48.1)
  line L249 (48.8929, 45.1929) -> (51.8, 48.1)
  arc A84 (57.4071, 46.2929) -> (58.1142, 46) centre (58.1142, 47) ccw
  arc A85 (58.1142, 54) -> (57.4071, 53.7071) centre (58.1142, 53) ccw
  line L250 (57.4071, 46.2929) -> (54.5, 49.2)
  line L251 (54.5, 50) -> (54.5, 50.8)
  line L252 (54.5, 50) -> (54.5, 49.2)
  line L253 (57.4071, 53.7071) -> (54.5, 50.8)
  line L254 (58.1142, 54) -> (100.8858, 54)
  line L255 (100.8858, 46) -> (58.1142, 46)
  arc A86 (101.5929, 53.7071) -> (100.8858, 54) centre (100.8858, 53) ccw
  arc A87 (100.8858, 46) -> (101.5929, 46.2929) centre (100.8858, 47) ccw
  line L256 (101.5929, 46.2929) -> (104.5, 49.2)
  line L257 (104.5, 50) -> (104.5, 49.2)
  line L258 (104.5, 50) -> (104.5, 50.8)
  line L259 (101.5929, 53.7071) -> (104.5, 50.8)
  arc A88 (40.8071, -52.7929) -> (41.1, -52.0858) centre (40.1, -52.0858) ccw
  arc A89 (33.1, -52.0858) -> (33.3929, -52.7929) centre (34.1, -52.0858) ccw
  line L260 (40.8071, -52.7929) -> (37.9, -55.7)
  line L261 (37.1, -55.7) -> (36.3, -55.7)
  line L262 (37.1, -55.7) -> (37.9, -55.7)
  line L263 (33.3929, -52.7929) -> (36.3, -55.7)
  line L264 (33.1, -52.0858) -> (33.1, -9.3142)
  line L265 (41.1, -9.3142) -> (41.1, -52.0858)
  arc A90 (33.3929, -8.6071) -> (33.1, -9.3142) centre (34.1, -9.3142) ccw
  arc A91 (41.1, -9.3142) -> (40.8071, -8.6071) centre (40.1, -9.3142) ccw
  line L266 (40.8071, -8.6071) -> (37.9, -5.7)
  line L267 (37.1, -5.7) -> (37.9, -5.7)
  line L268 (37.1, -5.7) -> (36.3, -5.7)
  line L269 (33.3929, -8.6071) -> (36.3, -5.7)
  arc A92 (-11.8929, -61.3071) -> (-11.1858, -61.6) centre (-11.1858, -60.6) ccw
  arc A93 (-11.1858, -53.6) -> (-11.8929, -53.8929) centre (-11.1858, -54.6) ccw
  line L270 (-11.8929, -61.3071) -> (-14.8, -58.4)
  line L271 (-14.8, -57.6) -> (-14.8, -56.8)
  line L272 (-14.8, -57.6) -> (-14.8, -58.4)
  line L273 (-11.8929, -53.8929) -> (-14.8, -56.8)
  line L274 (-11.1858, -53.6) -> (31.5858, -53.6)
  line L275 (31.5858, -61.6) -> (-11.1858, -61.6)
  arc A94 (32.2929, -53.8929) -> (31.5858, -53.6) centre (31.5858, -54.6) ccw
  arc A95 (31.5858, -61.6) -> (32.2929, -61.3071) centre (31.5858, -60.6) ccw
  line L276 (32.2929, -61.3071) -> (35.2, -58.4)
  line L277 (35.2, -57.6) -> (35.2, -58.4)
  line L278 (35.2, -57.6) -> (35.2, -56.8)
  line L279 (32.2929, -53.8929) -> (35.2, -56.8)
  arc A96 (-12.9929, -52.7929) -> (-12.7, -52.0858) centre (-13.7, -52.0858) ccw
  arc A97 (-20.7, -52.0858) -> (-20.4071, -52.7929) centre (-19.7, -52.0858) ccw
  line L280 (-12.9929, -52.7929) -> (-15.9, -55.7)
  line L281 (-16.7, -55.7) -> (-17.5, -55.7)
  line L282 (-16.7, -55.7) -> (-15.9, -55.7)
  line L283 (-20.4071, -52.7929) -> (-17.5, -55.7)
  line L284 (-20.7, -52.0858) -> (-20.7, -9.3142)
  line L285 (-12.7, -9.3142) -> (-12.7, -52.0858)
  arc A98 (-20.4071, -8.6071) -> (-20.7, -9.3142) centre (-19.7, -9.3142) ccw
  arc A99 (-12.7, -9.3142) -> (-12.9929, -8.6071) centre (-13.7, -9.3142) ccw
  line L286 (-12.9929, -8.6071) -> (-15.9, -5.7)
  line L287 (-16.7, -5.7) -> (-15.9, -5.7)
  line L288 (-16.7, -5.7) -> (-17.5, -5.7)
  line L289 (-20.4071, -8.6071) -> (-17.5, -5.7)
  arc A100 (40.8071, 1.0071) -> (41.1, 1.7142) centre (40.1, 1.7142) ccw
  arc A101 (33.1, 1.7142) -> (33.3929, 1.0071) centre (34.1, 1.7142) ccw
  line L290 (40.8071, 1.0071) -> (37.9, -1.9)
  line L291 (37.1, -1.9) -> (36.3, -1.9)
  line L292 (37.1, -1.9) -> (37.9, -1.9)
  line L293 (33.3929, 1.0071) -> (36.3, -1.9)
  line L294 (33.1, 1.7142) -> (33.1, 44.4858)
  line L295 (41.1, 44.4858) -> (41.1, 1.7142)
  arc A102 (33.3929, 45.1929) -> (33.1, 44.4858) centre (34.1, 44.4858) ccw
  arc A103 (41.1, 44.4858) -> (40.8071, 45.1929) centre (40.1, 44.4858) ccw
  line L296 (40.8071, 45.1929) -> (37.9, 48.1)
  line L297 (37.1, 48.1) -> (37.9, 48.1)
  line L298 (37.1, 48.1) -> (36.3, 48.1)
  line L299 (33.3929, 45.1929) -> (36.3, 48.1)
  arc A104 (-11.8929, -7.5071) -> (-11.1858, -7.8) centre (-11.1858, -6.8) ccw
  arc A105 (-11.1858, 0.2) -> (-11.8929, -0.0929) centre (-11.1858, -0.8) ccw
  line L300 (-11.8929, -7.5071) -> (-14.8, -4.6)
  line L301 (-14.8, -3.8) -> (-14.8, -3)
  line L302 (-14.8, -3.8) -> (-14.8, -4.6)
  line L303 (-11.8929, -0.0929) -> (-14.8, -3)
  line L304 (-11.1858, 0.2) -> (31.5858, 0.2)
  line L305 (31.5858, -7.8) -> (-11.1858, -7.8)
  arc A106 (32.2929, -0.0929) -> (31.5858, 0.2) centre (31.5858, -0.8) ccw
  arc A107 (31.5858, -7.8) -> (32.2929, -7.5071) centre (31.5858, -6.8) ccw
  line L306 (32.2929, -7.5071) -> (35.2, -4.6)
  line L307 (35.2, -3.8) -> (35.2, -4.6)
  line L308 (35.2, -3.8) -> (35.2, -3)
  line L309 (32.2929, -0.0929) -> (35.2, -3)
  arc A108 (-12.9929, 1.0071) -> (-12.7, 1.7142) centre (-13.7, 1.7142) ccw
  arc A109 (-20.7, 1.7142) -> (-20.4071, 1.0071) centre (-19.7, 1.7142) ccw
  line L310 (-12.9929, 1.0071) -> (-15.9, -1.9)
  line L311 (-16.7, -1.9) -> (-17.5, -1.9)
  line L312 (-16.7, -1.9) -> (-15.9, -1.9)
  line L313 (-20.4071, 1.0071) -> (-17.5, -1.9)
  line L314 (-20.7, 1.7142) -> (-20.7, 44.4858)
  line L315 (-12.7, 44.4858) -> (-12.7, 1.7142)
  arc A110 (-20.4071, 45.1929) -> (-20.7, 44.4858) centre (-19.7, 44.4858) ccw
  arc A111 (-12.7, 44.4858) -> (-12.9929, 45.1929) centre (-13.7, 44.4858) ccw
  line L316 (-12.9929, 45.1929) -> (-15.9, 48.1)
  line L317 (-16.7, 48.1) -> (-15.9, 48.1)
  line L318 (-16.7, 48.1) -> (-17.5, 48.1)
  line L319 (-20.4071, 45.1929) -> (-17.5, 48.1)
  arc A112 (-11.8929, 46.2929) -> (-11.1858, 46) centre (-11.1858, 47) ccw
  arc A113 (-11.1858, 54) -> (-11.8929, 53.7071) centre (-11.1858, 53) ccw
  line L320 (-11.8929, 46.2929) -> (-14.8, 49.2)
  line L321 (-14.8, 50) -> (-14.8, 50.8)
  line L322 (-14.8, 50) -> (-14.8, 49.2)
  line L323 (-11.8929, 53.7071) -> (-14.8, 50.8)
  line L324 (-11.1858, 54) -> (31.5858, 54)
  line L325 (31.5858, 46) -> (-11.1858, 46)
  arc A114 (32.2929, 53.7071) -> (31.5858, 54) centre (31.5858, 53) ccw
  arc A115 (31.5858, 46) -> (32.2929, 46.2929) centre (31.5858, 47) ccw
  line L326 (32.2929, 46.2929) -> (35.2, 49.2)
  line L327 (35.2, 50) -> (35.2, 49.2)
  line L328 (35.2, 50) -> (35.2, 50.8)
  line L329 (32.2929, 53.7071) -> (35.2, 50.8)
  arc A116 (-45.9929, -52.7929) -> (-45.7, -52.0858) centre (-46.7, -52.0858) ccw
  arc A117 (-53.7, -52.0858) -> (-53.4071, -52.7929) centre (-52.7, -52.0858) ccw
  line L330 (-45.9929, -52.7929) -> (-48.9, -55.7)
  line L331 (-49.7, -55.7) -> (-50.5, -55.7)
  line L332 (-49.7, -55.7) -> (-48.9, -55.7)
  line L333 (-53.4071, -52.7929) -> (-50.5, -55.7)
  line L334 (-53.7, -52.0858) -> (-53.7, -9.3142)
  line L335 (-45.7, -9.3142) -> (-45.7, -52.0858)
  arc A118 (-53.4071, -8.6071) -> (-53.7, -9.3142) centre (-52.7, -9.3142) ccw
  arc A119 (-45.7, -9.3142) -> (-45.9929, -8.6071) centre (-46.7, -9.3142) ccw
  line L336 (-45.9929, -8.6071) -> (-48.9, -5.7)
  line L337 (-49.7, -5.7) -> (-48.9, -5.7)
  line L338 (-49.7, -5.7) -> (-50.5, -5.7)
  line L339 (-53.4071, -8.6071) -> (-50.5, -5.7)
  arc A120 (-98.6929, -61.3071) -> (-97.9858, -61.6) centre (-97.9858, -60.6) ccw
  arc A121 (-97.9858, -53.6) -> (-98.6929, -53.8929) centre (-97.9858, -54.6) ccw
  line L340 (-98.6929, -61.3071) -> (-101.6, -58.4)
  line L341 (-101.6, -57.6) -> (-101.6, -56.8)
  line L342 (-101.6, -57.6) -> (-101.6, -58.4)
  line L343 (-98.6929, -53.8929) -> (-101.6, -56.8)
  line L344 (-97.9858, -53.6) -> (-55.2142, -53.6)
  line L345 (-55.2142, -61.6) -> (-97.9858, -61.6)
  arc A122 (-54.5071, -53.8929) -> (-55.2142, -53.6) centre (-55.2142, -54.6) ccw
  arc A123 (-55.2142, -61.6) -> (-54.5071, -61.3071) centre (-55.2142, -60.6) ccw
  line L346 (-54.5071, -61.3071) -> (-51.6, -58.4)
  line L347 (-51.6, -57.6) -> (-51.6, -58.4)
  line L348 (-51.6, -57.6) -> (-51.6, -56.8)
  line L349 (-54.5071, -53.8929) -> (-51.6, -56.8)
  arc A124 (-99.7929, -52.7929) -> (-99.5, -52.0858) centre (-100.5, -52.0858) ccw
  arc A125 (-107.5, -52.0858) -> (-107.2071, -52.7929) centre (-106.5, -52.0858) ccw
  line L350 (-99.7929, -52.7929) -> (-102.7, -55.7)
  line L351 (-103.5, -55.7) -> (-104.3, -55.7)
  line L352 (-103.5, -55.7) -> (-102.7, -55.7)
  line L353 (-107.2071, -52.7929) -> (-104.3, -55.7)
  line L354 (-107.5, -52.0858) -> (-107.5, -9.3142)
  line L355 (-99.5, -9.3142) -> (-99.5, -52.0858)
  arc A126 (-107.2071, -8.6071) -> (-107.5, -9.3142) centre (-106.5, -9.3142) ccw
  arc A127 (-99.5, -9.3142) -> (-99.7929, -8.6071) centre (-100.5, -9.3142) ccw
  line L356 (-99.7929, -8.6071) -> (-102.7, -5.7)
  line L357 (-103.5, -5.7) -> (-102.7, -5.7)
  line L358 (-103.5, -5.7) -> (-104.3, -5.7)
  line L359 (-107.2071, -8.6071) -> (-104.3, -5.7)
  arc A128 (-45.9929, 1.0071) -> (-45.7, 1.7142) centre (-46.7, 1.7142) ccw
  arc A129 (-53.7, 1.7142) -> (-53.4071, 1.0071) centre (-52.7, 1.7142) ccw
  line L360 (-45.9929, 1.0071) -> (-48.9, -1.9)
  line L361 (-49.7, -1.9) -> (-50.5, -1.9)
  line L362 (-49.7, -1.9) -> (-48.9, -1.9)
  line L363 (-53.4071, 1.0071) -> (-50.5, -1.9)
  line L364 (-53.7, 1.7142) -> (-53.7, 44.4858)
  line L365 (-45.7, 44.4858) -> (-45.7, 1.7142)
  arc A130 (-53.4071, 45.1929) -> (-53.7, 44.4858) centre (-52.7, 44.4858) ccw
  arc A131 (-45.7, 44.4858) -> (-45.9929, 45.1929) centre (-46.7, 44.4858) ccw
  line L366 (-45.9929, 45.1929) -> (-48.9, 48.1)
  line L367 (-49.7, 48.1) -> (-48.9, 48.1)
  line L368 (-49.7, 48.1) -> (-50.5, 48.1)
  line L369 (-53.4071, 45.1929) -> (-50.5, 48.1)
  arc A132 (-98.6929, -7.5071) -> (-97.9858, -7.8) centre (-97.9858, -6.8) ccw
  arc A133 (-97.9858, 0.2) -> (-98.6929, -0.0929) centre (-97.9858, -0.8) ccw
  line L370 (-98.6929, -7.5071) -> (-101.6, -4.6)
  line L371 (-101.6, -3.8) -> (-101.6, -3)
  line L372 (-101.6, -3.8) -> (-101.6, -4.6)
  line L373 (-98.6929, -0.0929) -> (-101.6, -3)
  line L374 (-97.9858, 0.2) -> (-55.2142, 0.2)
  line L375 (-55.2142, -7.8) -> (-97.9858, -7.8)
  arc A134 (-54.5071, -0.0929) -> (-55.2142, 0.2) centre (-55.2142, -0.8) ccw
  arc A135 (-55.2142, -7.8) -> (-54.5071, -7.5071) centre (-55.2142, -6.8) ccw
  line L376 (-54.5071, -7.5071) -> (-51.6, -4.6)
  line L377 (-51.6, -3.8) -> (-51.6, -4.6)
  line L378 (-51.6, -3.8) -> (-51.6, -3)
  line L379 (-54.5071, -0.0929) -> (-51.6, -3)
  arc A136 (-99.7929, 1.0071) -> (-99.5, 1.7142) centre (-100.5, 1.7142) ccw
  arc A137 (-107.5, 1.7142) -> (-107.2071, 1.0071) centre (-106.5, 1.7142) ccw
  line L380 (-99.7929, 1.0071) -> (-102.7, -1.9)
  line L381 (-103.5, -1.9) -> (-104.3, -1.9)
  line L382 (-103.5, -1.9) -> (-102.7, -1.9)
  line L383 (-107.2071, 1.0071) -> (-104.3, -1.9)
  line L384 (-107.5, 1.7142) -> (-107.5, 44.4858)
  line L385 (-99.5, 44.4858) -> (-99.5, 1.7142)
  arc A138 (-107.2071, 45.1929) -> (-107.5, 44.4858) centre (-106.5, 44.4858) ccw
  arc A139 (-99.5, 44.4858) -> (-99.7929, 45.1929) centre (-100.5, 44.4858) ccw
  line L386 (-99.7929, 45.1929) -> (-102.7, 48.1)
  line L387 (-103.5, 48.1) -> (-102.7, 48.1)
  line L388 (-103.5, 48.1) -> (-104.3, 48.1)
  line L389 (-107.2071, 45.1929) -> (-104.3, 48.1)
  arc A140 (-98.6929, 46.2929) -> (-97.9858, 46) centre (-97.9858, 47) ccw
  arc A141 (-97.9858, 54) -> (-98.6929, 53.7071) centre (-97.9858, 53) ccw
  line L390 (-98.6929, 46.2929) -> (-101.6, 49.2)
  line L391 (-101.6, 50) -> (-101.6, 50.8)
  line L392 (-101.6, 50) -> (-101.6, 49.2)
  line L393 (-98.6929, 53.7071) -> (-101.6, 50.8)
  line L394 (-97.9858, 54) -> (-55.2142, 54)
  line L395 (-55.2142, 46) -> (-97.9858, 46)
  arc A142 (-54.5071, 53.7071) -> (-55.2142, 54) centre (-55.2142, 53) ccw
  arc A143 (-55.2142, 46) -> (-54.5071, 46.2929) centre (-55.2142, 47) ccw
  line L396 (-54.5071, 46.2929) -> (-51.6, 49.2)
  line L397 (-51.6, 50) -> (-51.6, 49.2)
  line L398 (-51.6, 50) -> (-51.6, 50.8)
  line L399 (-54.5071, 53.7071) -> (-51.6, 50.8)
  arc A144 (-115.2929, -52.7929) -> (-115, -52.0858) centre (-116, -52.0858) ccw
  arc A145 (-123, -52.0858) -> (-122.7071, -52.7929) centre (-122, -52.0858) ccw
  line L400 (-115.2929, -52.7929) -> (-118.2, -55.7)
  line L401 (-119, -55.7) -> (-119.8, -55.7)
  line L402 (-119, -55.7) -> (-118.2, -55.7)
  line L403 (-122.7071, -52.7929) -> (-119.8, -55.7)
  line L404 (-123, -52.0858) -> (-123, -9.3142)
  line L405 (-115, -9.3142) -> (-115, -52.0858)
  arc A146 (-122.7071, -8.6071) -> (-123, -9.3142) centre (-122, -9.3142) ccw
  arc A147 (-115, -9.3142) -> (-115.2929, -8.6071) centre (-116, -9.3142) ccw
  line L406 (-115.2929, -8.6071) -> (-118.2, -5.7)
  line L407 (-119, -5.7) -> (-118.2, -5.7)
  line L408 (-119, -5.7) -> (-119.8, -5.7)
  line L409 (-122.7071, -8.6071) -> (-119.8, -5.7)
  arc A148 (-167.9929, -61.3071) -> (-167.2858, -61.6) centre (-167.2858, -60.6) ccw
  arc A149 (-167.2858, -53.6) -> (-167.9929, -53.8929) centre (-167.2858, -54.6) ccw
  line L410 (-167.9929, -61.3071) -> (-170.9, -58.4)
  line L411 (-170.9, -57.6) -> (-170.9, -56.8)
  line L412 (-170.9, -57.6) -> (-170.9, -58.4)
  line L413 (-167.9929, -53.8929) -> (-170.9, -56.8)
  line L414 (-167.2858, -53.6) -> (-124.5142, -53.6)
  line L415 (-124.5142, -61.6) -> (-167.2858, -61.6)
  arc A150 (-123.8071, -53.8929) -> (-124.5142, -53.6) centre (-124.5142, -54.6) ccw
  arc A151 (-124.5142, -61.6) -> (-123.8071, -61.3071) centre (-124.5142, -60.6) ccw